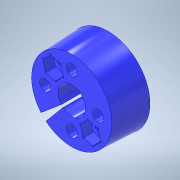
# Autodesk Inventor part: TimingPulley_S5M_MechaLock_2
Saved by Autodesk Inventor 2022 (Build 260153000, 153)
## iProperties
Created: 2022-03-19
Part Number: TimingPulley_S5M_MechaLock_2
Material: ABS プラスチック
Document SubType Name: Modeling
Designer: satot
Density: 1.06 g/cm^3
Appearance: 青 - 壁塗料 - 光沢
Author: satot
Autodesk Inventor part; units mm, degrees
ref_plane "XZ Plane" through (0, 0, 0) normal (0, 1, 0) x (-1, 0, 0)
ref_plane "XY Plane" through (0, 0, 0) normal (0, 0, 1) x (1, 0, 0)
sketch "スケッチ1" plane through (0, 0, 0) normal (1, 0, 0) x (0, 1, 0)
  circle A0 centre (0, 0) radius 12.6
  dimension "d0" = 25.2
  constraints: 1 centre point, 1 coincident
  measures "d0" diameter of A0
ref_plane "作業平面1" through (11, 0, 0) normal (1, 0, 0) x (0, 1, 0)
sketch "スケッチ2" plane through (11, 0, 0) normal (1, 0, 0) x (0, 1, 0)
  circle A0 centre (0, 0) radius 12.1188
  dimension "d2" = 24.2376
  constraints: 1 centre point, 1 coincident
  measures "d2" diameter of A0
loft "ロフト1" add profiles "スケッチ1", "スケッチ2"
sketch "スケッチ3" plane through (0, 0, 0) normal (-1, 0, 0) x (0, 0, 1)
  point P0 (0, 0)
  point P1 (0, 0)
  constraints: 1 coincident
hole "穴1" at (0, 0, 0) direction (1, 0, 0) diameter 8.3 end through all
sketch "スケッチ4" plane through (0, 0, 0) normal (-1, 0, 0) x (0, 0, 1)
  point P0 (0, 0)
  point P1 (0, 8)
  point P2 (-8, 0)
  point P3 (0, -8)
  point P4 (8, 0)
  dimension "d14" = 8
  dimension "d17" = 360
  constraints: 1 vertical alignment, 5 other
  measures "d14" distance of point (0, 0) point (0, 8)
hole "穴2" at (0, 8, 0) at (0, 0, -8) at (0, -8, 0) at (0, 0, 8) direction (1, 0, 0) diameter 3.4 end through all
sketch "スケッチ5" plane through (0, 0, 0) normal (-1, 0, 0) x (0, 0, 1)
  circle A0 centre (0, -8) radius 1.7 projected
  line L0 (3.2332, -8) -> (1.6166, -10.8)
  line L1 (1.6166, -10.8) -> (-1.6166, -10.8)
  line L2 (-1.6166, -10.8) -> (-3.2332, -8)
  line L3 (-3.2332, -8) -> (-1.6166, -5.2)
  line L4 (-1.6166, -5.2) -> (1.6166, -5.2)
  line L5 (1.6166, -5.2) -> (3.2332, -8)
  circle A1 centre (-1.6166, -10.8) radius 0.2
  circle A2 centre (1.6166, -10.8) radius 0.2
  circle A3 centre (3.2332, -8) radius 0.2
  circle A4 centre (1.6166, -5.2) radius 0.2
  circle A5 centre (-1.6166, -5.2) radius 0.2
  circle A6 centre (-3.2332, -8) radius 0.2
  circle A7 centre (5.2, -1.6166) radius 0.2
  line L6 (5.2, -1.6166) -> (5.2, 1.6166)
  line L7 (5.2, 1.6166) -> (8, 3.2332)
  circle A8 centre (8, 3.2332) radius 0.2
  line L8 (8, -3.2332) -> (5.2, -1.6166)
  circle A9 centre (8, -3.2332) radius 0.2
  line L9 (8, 3.2332) -> (10.8, 1.6166)
  circle A10 centre (10.8, 1.6166) radius 0.2
  line L10 (10.8, 1.6166) -> (10.8, -1.6166)
  circle A11 centre (10.8, -1.6166) radius 0.2
  line L11 (10.8, -1.6166) -> (8, -3.2332)
  circle A12 centre (5.2, 1.6166) radius 0.2
  circle A13 centre (1.6166, 5.2) radius 0.2
  line L12 (1.6166, 5.2) -> (-1.6166, 5.2)
  line L13 (-1.6166, 5.2) -> (-3.2332, 8)
  circle A14 centre (-3.2332, 8) radius 0.2
  line L14 (3.2332, 8) -> (1.6166, 5.2)
  circle A15 centre (3.2332, 8) radius 0.2
  line L15 (-3.2332, 8) -> (-1.6166, 10.8)
  circle A16 centre (-1.6166, 10.8) radius 0.2
  line L16 (-1.6166, 10.8) -> (1.6166, 10.8)
  circle A17 centre (1.6166, 10.8) radius 0.2
  line L17 (1.6166, 10.8) -> (3.2332, 8)
  circle A18 centre (-1.6166, 5.2) radius 0.2
  circle A19 centre (-5.2, 1.6166) radius 0.2
  line L18 (-5.2, 1.6166) -> (-5.2, -1.6166)
  line L19 (-5.2, -1.6166) -> (-8, -3.2332)
  circle A20 centre (-8, -3.2332) radius 0.2
  line L20 (-8, 3.2332) -> (-5.2, 1.6166)
  circle A21 centre (-8, 3.2332) radius 0.2
  line L21 (-8, -3.2332) -> (-10.8, -1.6166)
  circle A22 centre (-10.8, -1.6166) radius 0.2
  line L22 (-10.8, -1.6166) -> (-10.8, 1.6166)
  circle A23 centre (-10.8, 1.6166) radius 0.2
  line L23 (-10.8, 1.6166) -> (-8, 3.2332)
  circle A24 centre (-5.2, -1.6166) radius 0.2
  point P0 (0, 0)
  point P1 (8, 0)
  point P2 (8, 0)
  point P3 (8, 0)
  point P4 (8, 0)
  point P5 (8, 0)
  point P6 (8, 0)
  point P7 (8, 0)
  point P8 (0, 8)
  point P9 (0, 8)
  point P10 (0, 8)
  point P11 (0, 8)
  point P12 (0, 8)
  point P13 (0, 8)
  point P14 (0, 8)
  point P15 (-8, 0)
  point P16 (-8, 0)
  point P17 (-8, 0)
  point P18 (-8, 0)
  point P19 (-8, 0)
  point P20 (-8, 0)
  point P21 (-8, 0)
  point P22 (-5.2, -1.4166)
  point P23 (-5.2, 1.4166)
  point P24 (-5.3732, 1.7166)
  point P25 (-7.8268, 3.1332)
  point P26 (-8.1732, 3.1332)
  point P27 (-10.6268, 1.7166)
  point P28 (-10.8, 1.4166)
  point P29 (-10.8, -1.4166)
  point P30 (-10.6268, -1.7166)
  point P31 (-8.1732, -3.1332)
  point P32 (-7.8268, -3.1332)
  point P33 (-5.3732, -1.7166)
  point P34 (-1.4166, 5.2)
  point P35 (1.4166, 5.2)
  point P36 (1.7166, 5.3732)
  point P37 (3.1332, 7.8268)
  point P38 (3.1332, 8.1732)
  point P39 (1.7166, 10.6268)
  point P40 (1.4166, 10.8)
  point P41 (-1.4166, 10.8)
  point P42 (-1.7166, 10.6268)
  point P43 (-3.1332, 8.1732)
  point P44 (-3.1332, 7.8268)
  point P45 (-1.7166, 5.3732)
  point P46 (5.2, 1.4166)
  point P47 (5.2, -1.4166)
  point P48 (5.3732, -1.7166)
  point P49 (7.8268, -3.1332)
  point P50 (8.1732, -3.1332)
  point P51 (10.6268, -1.7166)
  point P52 (10.8, -1.4166)
  point P53 (10.8, 1.4166)
  point P54 (10.6268, 1.7166)
  point P55 (8.1732, 3.1332)
  point P56 (7.8268, 3.1332)
  point P57 (5.3732, 1.7166)
  point P58 (-1.4166, -5.2)
  point P59 (-1.7166, -5.3732)
  point P60 (-3.1332, -7.8268)
  point P61 (-3.1332, -8.1732)
  point P62 (-1.7166, -10.6268)
  point P63 (-1.4166, -10.8)
  point P64 (1.7166, -10.6268)
  point P65 (1.4166, -10.8)
  point P66 (3.1332, -7.8268)
  point P67 (3.1332, -8.1732)
  point P68 (1.4166, -5.2)
  point P69 (1.7166, -5.3732)
  dimension "d26" = 5.6
  dimension "d62" = 0.4
  dimension "d65" = 360
  dimension "d73" = 360
  constraints: 48 end point, 24 centre point, 10 coincident, 1 horizontal alignment, 155 other
  measures "d26" distance between parallel lines of L4 L1
  measures "d62" diameter of A1
extrude "押し出し1" cut sketch "スケッチ5" against normal blind 3 contours A0 | L5 A3 L0 | L0 A3 L5 | L0 A2 L1 A1 L2 A6 L3 A5 L4 A4 L5 A3 | A2 L1 L0 | L0 L1 A2 | A4 L4 L5 | L5 L4 A4 | A1 L2 L1 | L1 L2 A1 | A5 L3 L4 | L4 L3 A5 | A6 L3 L2 | L2 L3 A6 | A7 L8 L6 | A7 L6 A12 L7 A8 L9 A10 L10 A11 L11 A9 L8 | L6 L8 A7 | A12 L7 L6 | L6 L7 A12 | A9 L11 L8 | L8 L11 A9 | A8 L9 L7 | L7 L9 A8 | L11 L10 A11 | A11 L10 L11 | A10 L10 L9 | L9 L10 A10 | A13 L12 L14 | L14 L12 A13 | A13 L12 A18 L13 A14 L15 A16 L16 A17 L17 A15 L14 | A15 L17 L14 | L14 L17 A15 | A18 L13 L12 | L12 L13 A18 | L17 L16 A17 | A17 L16 L17 | A14 L15 L13 | L13 L15 A14 | L16 L15 A16 | A16 L15 L16 | A19 L18 L20 | L20 L18 A19 | A19 L18 A24 L19 A20 L21 A22 L22 A23 L23 A21 L20 | A21 L23 L20 | L20 L23 A21 | A24 L19 L18 | L18 L19 A24 | L23 L22 A23 | A23 L22 L23 | A20 L21 L19 | L19 L21 A20 | L22 L21 A22 | A22 L21 L22
sketch "スケッチ6" plane through (0, 0, 0) normal (-1, 0, 0) x (0, 0, 1)
  line L0 (0, 0) -> (-8.0991, -9.6522)
  circle A0 centre (0, 0) radius 12.6 projected
  line L1 (-9.6522, -8.0991) -> (0, 0)
  line L2 (-9.6522, -8.0991) -> (-8.0991, -9.6522) construction
  line L3 (-8.8756, -8.8756) -> (0, 0) construction
  line L4 (0, -12.6) -> (0, 0) construction
  dimension "d33" = 45
  dimension "d34" = 10
  constraints: 10 end point, 3 point on circle, 1 midpoint, 1 vertical
  measures "d33" angle of L4 L3
  measures "d34" angle of L1 L0
extrude "押し出し2" cut sketch "スケッチ6" against normal through all contours L0 A0 L1 picked at (-6.2724, -5.5819)
sketch "スケッチ7" plane through (0, 0, 0) normal (-1, 0, 0) x (0, 0.7071068, 0.7071068)
  point P0 (0, 0)
  point P1 (0, -8)
  point P2 (0, 8)
  dimension "d37" = 8
  dimension "d40" = 360
  constraints: 1 vertical alignment, 3 other
  measures "d37" distance of point (0, -8) point (0, 0)
hole "穴3" at (0, -5.6569, 5.6569) at (0, 5.6569, -5.6569) direction (1, 0, 0) diameter 3.4 end through all
sketch "スケッチ8" plane through (11, 0, 0) normal (1, 0, 0) x (0, -0.7071068, -0.7071068)
  circle A0 centre (0, -8) radius 1.7 projected
  line L0 (-3.2332, -8) -> (-1.6166, -5.2)
  line L1 (-1.6166, -5.2) -> (1.6166, -5.2)
  line L2 (1.6166, -5.2) -> (3.2332, -8)
  line L3 (3.2332, -8) -> (1.6166, -10.8)
  line L4 (1.6166, -10.8) -> (-1.6166, -10.8)
  line L5 (-1.6166, -10.8) -> (-3.2332, -8)
  circle A1 centre (-3.2332, -8) radius 0.2
  circle A2 centre (-1.6166, -10.8) radius 0.2
  circle A3 centre (1.6166, -10.8) radius 0.2
  circle A4 centre (3.2332, -8) radius 0.2
  circle A5 centre (1.6166, -5.2) radius 0.2
  circle A6 centre (-1.6166, -5.2) radius 0.2
  circle A7 centre (1.6166, 10.8) radius 0.2
  line L6 (-1.6166, 10.8) -> (1.6166, 10.8)
  line L7 (1.6166, 10.8) -> (3.2332, 8)
  circle A8 centre (-1.6166, 10.8) radius 0.2
  circle A9 centre (3.2332, 8) radius 0.2
  line L8 (-3.2332, 8) -> (-1.6166, 10.8)
  circle A10 centre (-3.2332, 8) radius 0.2
  line L9 (1.6166, 5.2) -> (-1.6166, 5.2)
  circle A11 centre (-1.6166, 5.2) radius 0.2
  line L10 (-1.6166, 5.2) -> (-3.2332, 8)
  line L11 (3.2332, 8) -> (1.6166, 5.2)
  circle A12 centre (1.6166, 5.2) radius 0.2
  point P0 (0, 0)
  point P1 (0, 8)
  point P2 (0, 8)
  point P3 (0, 8)
  point P4 (0, 8)
  point P5 (0, 8)
  point P6 (0, 8)
  point P7 (0, 8)
  point P8 (-1.7166, -10.6268)
  point P9 (-1.4166, -10.8)
  point P10 (1.4166, -10.8)
  point P11 (1.7166, -10.6268)
  point P12 (3.1332, -7.8268)
  point P13 (3.1332, -8.1732)
  point P14 (1.4166, -5.2)
  point P15 (1.7166, -5.3732)
  point P16 (-1.4166, -5.2)
  point P17 (-1.7166, -5.3732)
  point P18 (-3.1332, -7.8268)
  point P19 (-3.1332, -8.1732)
  point P20 (3.1332, 7.8268)
  point P21 (3.1332, 8.1732)
  point P22 (1.7166, 5.3732)
  point P23 (1.7166, 10.6268)
  point P24 (1.4166, 10.8)
  point P25 (-1.4166, 10.8)
  point P26 (-1.7166, 10.6268)
  point P27 (-3.1332, 8.1732)
  point P28 (-3.1332, 7.8268)
  point P29 (-1.7166, 5.3732)
  point P30 (-1.4166, 5.2)
  point P31 (1.4166, 5.2)
  dimension "d50" = 5.6
  dimension "d53" = 0.4
  dimension "d56" = 360
  dimension "d60" = 360
  constraints: 24 end point, 12 centre point, 6 coincident, 1 horizontal alignment, 93 other
  measures "d50" distance between parallel lines of L3 L0
  measures "d53" diameter of A1
extrude "押し出し3" cut sketch "スケッチ8" against normal blind 3 contours L5 A1 L0 | L0 A1 L5 | L0 A6 L1 A5 L2 A4 L3 A3 L4 A2 L5 A1 | A6 L1 L0 | L0 L1 A6 | A2 L4 L5 | L5 L4 A2 | A5 L2 L1 | L1 L2 A5 | A3 L3 L4 | L4 L3 A3 | A4 L3 L2 | L2 L3 A4 | A7 L7 L6 | L6 L7 A7 | A7 L7 A9 L11 A12 L9 A11 L10 A10 L8 A8 L6 | A8 L8 L6 | L6 L8 A8 | A9 L11 L7 | A10 L10 L8 | L8 L10 A10 | A12 L9 L11 | L11 L9 A12 | L10 L9 A11 | A11 L9 L10 picked at (3.3241, 8.0963)
equation "\"d7\" = 穴径"
equation "\"穴径\" = 8.3"
